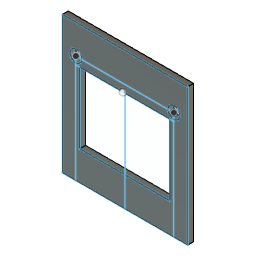
placa_baixo (Autodesk Fusion 360 design; units mm, degrees)
part number: 2025-10-18-19-38-59-563
Autodesk Fusion 360 part; units mm, degrees
sketch "Sketch9" plane through (0, 0, 0) normal (0, 1, 0) x (1, 0, 0)
  line L0 (-6, 8.1973) -> (26, 8.1973)
  line L1 (26, 8.1973) -> (26, -26.8027)
  line L2 (26, -26.8027) -> (-6, -26.8027)
  line L3 (-6, -26.8027) -> (-6, 8.1973)
  line L4 (10, 8.1973) -> (10, -17.3027)
  line L5 (22.4349, 8.1973) -> (22.4349, -19.3027)
  line L6 (-2.5651, 8.1973) -> (-2.5651, -19.3027)
  circle A0 centre (-2.5651, -19.3027) radius 1.5
  circle A1 centre (22.4349, -19.3027) radius 1.5
  line L7 (-2.5651, -19.3027) -> (22.4349, -19.3027)
  line L8 (10, -17.3027) -> (9.4349, -17.3027)
  line L9 (-2.5651, -17.35) -> (22.4349, -17.35)
  line L10 (9.9349, 0.6973) -> (-1.5651, 0.6973)
  line L11 (9.9349, 0.6973) -> (21.4349, 0.6973)
  line L12 (-1.5651, 0.6973) -> (-1.5651, -17.35)
  line L13 (21.4349, 0.6973) -> (21.4349, -17.35)
  dimension "d91" = 35
  dimension "d92" = 32
  dimension "d124" = 25.5
  dimension "d125" = 27.5
  dimension "d129" = 27.5
  dimension "d130" = 3
  dimension "d131" = 3
  dimension "d132" = 25
  dimension "d134" = 11.5
  dimension "d135" = 11.5
  constraint horizontal L0
  constraint vertical L1
  constraint horizontal L2
  constraint vertical L3
  constraint midpoint L0 L4.start
  constraint perpendicular L0 L4
  constraint coincident L0 L5.start
  constraint coincident L0 L6.start
  constraint coincident L6.end A0.centre
  constraint coincident L5.end A1.centre
  constraint perpendicular L4 L8
  constraint coincident L6 L9.start
  constraint coincident L5 L9.end
  constraint perpendicular L5 L9
  constraint coincident L9 L12.end
  constraint perpendicular L9 L12
  constraint coincident L9 L13.end
  constraint perpendicular L9 L13
  measures "d91" distance of L0.end L1.end
  measures "d92" distance of L0.start L0.end
  measures "d124" distance of L4.start L4.end
  measures "d125" distance of L5.start L5.end
  measures "d129" distance of L6.start L6.end
  measures "d130" diameter of A0
  measures "d131" diameter of A1
  measures "d132" distance of L5.end L6.end
  measures "d134" distance of L10.start L10.end
  measures "d135" distance of L10.start L11.end
extrude "Extrude15" add sketch "Sketch9" along normal blind 1.5 contours L0 L1 L2 L3 L5 L6 A0 A1 L7 | L0 L4 L6 L9 L10 L11 L12 | L0 L4 L5 L9 L11 L13 | L5 L6 A0 A1 L7 L9
